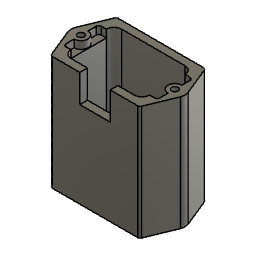
move_base_psd_holder (Autodesk Fusion 360 design; units mm, degrees)
Autodesk Fusion 360 part; units mm, degrees
note: some values were not read from the file. Set by a fixed rule: which sketch regions a step uses; the direction of a hole.
sketch "スケッチ1" plane through (0, 0, 0) normal (0, 1, 0) x (1, 0, 0)
  line L0 (17.5, 13) -> (-17.5, 13)
  line L1 (-17.5, 13) -> (-17.5, -13)
  line L2 (-17.5, -13) -> (17.5, -13)
  line L3 (17.5, -13) -> (17.5, 13)
  line L4 (17.5, 13) -> (-17.5, -13) construction
  line L5 (-17.5, 13) -> (17.5, -13) construction
  line L6 (-18.5, 0) -> (18.5, 0)
  circle A0 centre (-18.5, 0) radius 4
  circle A1 centre (18.5, 0) radius 4
  line L7 (17.5, 13) -> (22.2018, 1.5155)
  line L8 (17.5, -13) -> (22.2018, -1.5155)
  line L9 (-17.5, 13) -> (-22.2018, 1.5155)
  line L10 (-17.5, -13) -> (-22.2018, -1.5155)
  dimension "d3" = 26
  dimension "d4" = 35
  dimension "d5" = 37
  dimension "d6" = 8
  constraint horizontal L0
  constraint perpendicular L0 L1
  constraint parallel L0 L2
  constraint parallel L1 L3
  constraint coincident L4 origin
  constraint coincident L5 origin
  constraint horizontal L6
  constraint midpoint origin L6
  constraint coincident L6.start A0.centre
  constraint coincident L6.end A1.centre
  constraint equal A0 A1
  constraint coincident A1 L7.end
  constraint coincident A1 L8.end
  constraint coincident A0 L9.end
  constraint coincident A0 L10.end
  constraint tangent A0 L10
  constraint tangent A0 L9
  constraint tangent A1 L7
  constraint tangent A1 L8
  measures "d3" distance of L0.end L1.end
  measures "d4" distance of L0.start L0.end
  measures "d5" distance of L6.start L6.end
  measures "d6" diameter of A1
extrude "押し出し1" add sketch "スケッチ1" along normal blind 45
hole "穴1" at (-18.5, 0, 0) at (18.5, 0, 0) direction (0, 1, 0) diameter 2.5 end through all
sketch "スケッチ2" plane through (0, 0, 0) normal (0, -1, 0) x (1, 0, 0)
  circle A0 centre (-18.5, 0) radius 1.25
  circle A1 centre (18.5, 0) radius 1.25
  line L0 (22.2018, 1.5155) -> (17.5, 13)
  line L1 (17.5, 13) -> (-17.5, 13)
  line L2 (-17.5, 13) -> (-22.2018, 1.5155)
  arc A2 (-22.2018, 1.5155) -> (-22.2018, -1.5155) centre (-18.5, 0) ccw
  line L3 (-22.2018, -1.5155) -> (-17.5, -13)
  line L4 (-17.5, -13) -> (17.5, -13)
  line L5 (17.5, -13) -> (22.2018, -1.5155)
  arc A3 (22.2018, -1.5155) -> (22.2018, 1.5155) centre (18.5, 0) ccw
  line L6 (15.5, 10) -> (-15.5, 10)
  line L7 (-15.5, 10) -> (-15.5, -10)
  line L8 (-15.5, -10) -> (15.5, -10)
  line L9 (15.5, -10) -> (15.5, 10)
  line L10 (15.5, 10) -> (-15.5, -10) construction
  line L11 (-15.5, 10) -> (15.5, -10) construction
  dimension "d12" = 31
  dimension "d13" = 20
  constraint horizontal L6
  constraint perpendicular L6 L7
  constraint parallel L6 L8
  constraint parallel L7 L9
  constraint coincident L10 origin
  constraint coincident L11 origin
  measures "d12" distance of L6.start L6.end
  measures "d13" distance of L6.end L7.end
extrude "押し出し2" cut sketch "スケッチ2" against normal through all contours L6 L7 L8 L9
sketch "スケッチ3" plane through (0, 45, 0) normal (0, 1, 0) x (-1, 0, 0)
  line L0 (15.5, -10) -> (-15.5, -10)
  line L1 (-15.5, -10) -> (-15.5, 10)
  line L2 (-15.5, 10) -> (15.5, 10)
  line L3 (15.5, 10) -> (15.5, -10)
  circle A0 centre (18.5, 0) radius 1.25
  circle A1 centre (-18.5, 0) radius 1.25
  line L4 (-17.5, 13) -> (-22.2018, 1.5155)
  arc A2 (-22.2018, 1.5155) -> (-22.2018, -1.5155) centre (-18.5, 0) ccw
  line L5 (-22.2018, -1.5155) -> (-17.5, -13)
  line L6 (-17.5, -13) -> (17.5, -13)
  line L7 (17.5, -13) -> (22.2018, -1.5155)
  arc A3 (22.2018, -1.5155) -> (22.2018, 1.5155) centre (18.5, 0) ccw
  line L8 (22.2018, 1.5155) -> (17.5, 13)
  line L9 (17.5, 13) -> (-17.5, 13)
  line L10 (-23, -7) -> (23, -7)
  line L11 (23, -7) -> (23, 7)
  line L12 (23, 7) -> (-23, 7)
  line L13 (-23, 7) -> (-23, -7)
  line L14 (-23, -7) -> (23, 7) construction
  line L15 (23, -7) -> (-23, 7) construction
  line L16 (-6, 15) -> (6, 15)
  line L17 (6, 15) -> (6, 7)
  line L18 (6, 7) -> (-6, 7)
  line L19 (-6, 7) -> (-6, 15)
  line L20 (-6, 15) -> (6, 7) construction
  line L21 (6, 15) -> (-6, 7) construction
  line L22 (18.5, 0) -> (-18.5, 0)
  circle A4 centre (-18.5, 0) radius 2.75
  circle A5 centre (18.5, 0) radius 2.75
  line L23 (18.5, -7) -> (18.5, 7)
  line L24 (-18.5, -7) -> (-18.5, 7)
  point P0 (0, 11)
  dimension "d15" = 14
  dimension "d16" = 46
  dimension "d17" = 12
  dimension "d18" = 8
  dimension "d27" = 37
  dimension "d28" = 5.5
  constraint horizontal L10
  constraint perpendicular L10 L11
  constraint parallel L10 L12
  constraint parallel L11 L13
  constraint coincident L14 origin
  constraint coincident L15 origin
  constraint horizontal L16
  constraint perpendicular L16 L17
  constraint parallel L16 L18
  constraint parallel L17 L19
  constraint coincident L20 P0
  constraint coincident L21 P0
  constraint vertical origin P0
  constraint coincident L12 L18.end
  constraint horizontal L22
  constraint midpoint origin L22
  constraint coincident A1.centre A2.centre
  constraint concentric A0 A5
  constraint equal A4 A5
  constraint coincident L10 L23.start
  constraint coincident L12 L23.end
  constraint perpendicular L12 L23
  constraint coincident L10 L24.start
  constraint coincident L12 L24.end
  constraint perpendicular L12 L24
  constraint coincident A1.centre L24
  constraint coincident A0.centre L23
  measures "d15" distance of L10.start L12.end
  measures "d16" distance of L10.start L10.end
  measures "d17" distance of L16.start L16.end
  measures "d18" distance of L16.end L17.end
  measures "d27" distance of A0.centre A1.centre
  measures "d28" diameter of A4
extrude "押し出し4" cut sketch "スケッチ3" against normal blind 11 contours L2 L9 L17 L19
fillet "フィレット1" radius 1 4 edges at (17.5, 22.5, 13) (-17.5, 22.5, 13) (17.5, 22.5, -13) (-17.5, 22.5, -13)
fillet "フィレット2" radius 3 4 edges at (-15.5, 22.5, 10) (15.5, 22.5, 10) (15.5, 22.5, -10) (-15.5, 22.5, -10)
extrude "押し出し5" cut sketch "スケッチ3" against normal blind 3 contours L3 L10 L22 A5 L23 | L1 L10 L22 A4 L24 | L3 L12 L22 A5 L23 | L1 L12 L22 A4 L24
fillet "フィレット3" radius 1 4 edges at (-18.5, 43.5, -7) (-18.5, 43.5, 7) (18.5, 43.5, 7) (18.5, 43.5, -7)
